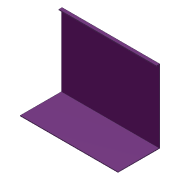
# Autodesk Inventor part: BatteryMount
Saved by Autodesk Inventor 2012 (Build 160160000, 160)
## iProperties
Created: 2013-02-01
Part Number: BatteryMount
Material: Aluminum-6061
Document SubType Name: Modeling
Designer: JesseK
Density: 2.71 g/cm^3
Mass: 290.438 g
Surface Area: 1372.17 cm^2
Volume: 107.173 cm^3
Author: JesseK
Autodesk Inventor part; units mm, degrees
ref_plane "YZ Plane" through (0, 0, 0) normal (1, 0, 0) x (0, 1, 0)
ref_plane "XZ Plane" through (0, 0, 0) normal (0, 1, 0) x (-1, 0, 0)
ref_plane "XY Plane" through (0, 0, 0) normal (0, 0, 1) x (1, 0, 0)
sketch "Sketch1" plane through (0, 0, 0) normal (1, 0, 0) x (0, 1, 0)
  line L0 (1.5875, 103.1875) -> (1.5875, 1.5875)
  line L1 (1.5875, 1.5875) -> (179.3875, 1.5875)
  line L2 (179.3875, 1.5875) -> (179.3875, 7.9375)
  line L3 (179.3875, 7.9375) -> (180.975, 7.9375)
  line L4 (180.975, 7.9375) -> (180.975, 0)
  line L5 (180.975, 0) -> (0, 0)
  line L6 (0, 0) -> (0, 103.1875)
  line L7 (0, 103.1875) -> (1.5875, 103.1875)
  dimension "d0" = 1.5875
  dimension "d1" = 1.5875
  dimension "d2" = 180.975
  dimension "d3" = 101.6
  dimension "d4" = 6.35
  constraints: 16 end point, 4 horizontal, 4 vertical, 1 parallel
  measures "d0" distance between parallel lines of L5 L1
  measures "d1" distance of L2.end L3.end
  measures "d2" distance of L4.end L5.end
  measures "d3" distance of L0.start L0.end
  measures "d4" distance of L1.end L2.end
extrude "Extrusion1" add sketch "Sketch1" along normal blind 241.3
sketch "Sketch2" plane through (0, 0, 0) normal (0, 0, -1) x (-1, 0, 0)
  line L0 (-241.3, 180.975) -> (-241.3, 0) projected
  line L1 (0, 0) -> (-241.3, 0) projected
  line L2 (0, 0) -> (0, 180.975) projected
  line L3 (-241.3, 127) -> (-215.9, 127)
  line L4 (-215.9, 127) -> (-215.9, 76.2)
  line L5 (-215.9, 76.2) -> (-241.3, 76.2)
  line L6 (-241.3, 76.2) -> (-241.3, 127)
  line L7 (0, 127) -> (-25.4, 127)
  line L8 (-25.4, 127) -> (-25.4, 76.2)
  line L9 (-25.4, 76.2) -> (0, 76.2)
  line L10 (0, 76.2) -> (0, 127)
  dimension "d7" = 25.4
  dimension "d8" = 50.8
  dimension "d9" = 76.2
  constraints: 16 end point, 4 parallel, 2 equal length, 2 horizontal, 2 perpendicular, 2 point on line, 1 collinear
  measures "d7" distance of L4.end L5.end
  measures "d8" distance of L3.end L4.end
  measures "d9" distance between parallel lines of L1 L5
extrude "Extrusion2" cut sketch "Sketch2" against normal up to next
sketch "Sketch3" plane through (0, 1.5875, 1.5875) normal (0, 0, 1) x (1, 0, 0)
  line L0 (0, 125.4125) -> (25.4, 125.4125) projected
  line L1 (241.3, 74.6125) -> (215.9, 74.6125) projected
  line L2 (215.9, 125.4125) -> (214.3125, 125.4125)
  line L3 (214.3125, 125.4125) -> (214.3125, 74.6125)
  line L4 (214.3125, 74.6125) -> (215.9, 74.6125)
  line L5 (215.9, 74.6125) -> (215.9, 125.4125)
  line L6 (25.4, 74.6125) -> (26.9875, 74.6125)
  line L7 (26.9875, 74.6125) -> (26.9875, 125.4125)
  line L8 (26.9875, 125.4125) -> (25.4, 125.4125)
  line L9 (25.4, 125.4125) -> (25.4, 74.6125)
  point P0 (0, -1.5875)
  dimension "d12" = 1.5875
  constraints: 16 end point, 4 parallel, 3 collinear, 2 horizontal, 2 perpendicular
  measures "d12" distance of L3.end L4.end
extrude "Extrusion3" add sketch "Sketch3" along normal blind 25.4
sketch "Sketch4" plane through (0, 179.3875, 1.5875) normal (0, 0, 1) x (1, 0, 0)
  line L0 (0, 0) -> (0, -52.3875) projected
  line L1 (241.3, -177.8) -> (241.3, -103.1875) projected
  circle A0 centre (228.6, -23.8125) radius 3.1877
  circle A1 centre (228.6, -125.4125) radius 3.1877
  circle A2 centre (12.7, -23.8125) radius 3.1877
  circle A3 centre (12.7, -125.4125) radius 3.1877
  line L2 (12.7, -23.8125) -> (228.6, -23.8125) construction
  line L3 (228.6, -23.8125) -> (228.6, -125.4125) construction
  line L4 (228.6, -125.4125) -> (12.7, -125.4125) construction
  line L5 (12.7, -125.4125) -> (12.7, -23.8125) construction
  line L6 (0, -179.3875) -> (241.3, -179.3875) construction
  line L7 (0, 1.5875) -> (241.3, 1.5875) construction
  dimension "d15" = 6.3754
  dimension "d16" = 12.7
  dimension "d18" = 25.4
  dimension "d19" = 101.6
  dimension "d20" = 12.7
  constraints: 8 end point, 4 centre point, 3 equal radius, 2 coincident, 2 parallel, 1 horizontal, 1 perpendicular
  measures "d15" diameter of A1
  measures "d16" distance between parallel lines of L0 L5
  measures "d18" distance between parallel lines of L7 L2
  measures "d19" distance of L4.end L2.start
  measures "d20" distance between parallel lines of L1 L3
extrude "Extrusion4" cut sketch "Sketch4" against normal through all
sketch "Sketch5" plane through (0, 0, 0) normal (0, -1, 0) x (1, 0, 0)
  line L0 (0, 103.1875) -> (31.75, 103.1875)
  line L1 (31.75, 103.1875) -> (31.75, 71.4375)
  line L2 (31.75, 71.4375) -> (0, 71.4375)
  line L3 (0, 71.4375) -> (0, 103.1875)
  line L4 (241.3, 103.1875) -> (209.55, 103.1875)
  line L5 (209.55, 103.1875) -> (209.55, 71.4375)
  line L6 (209.55, 71.4375) -> (241.3, 71.4375)
  line L7 (241.3, 71.4375) -> (241.3, 103.1875)
  dimension "d23" = 31.75
  constraints: 16 end point, 4 parallel, 3 equal length, 2 horizontal, 2 perpendicular
  measures "d23" distance between parallel lines of L3 L1
extrude "Extrusion5" cut sketch "Sketch5" against normal up to next
sketch "Sketch6" plane through (0, 1.5875, 1.5875) normal (0, 1, 0) x (1, 0, 0)
  line L0 (209.55, -101.6) -> (209.55, -69.85) projected
  line L1 (31.75, -69.85) -> (31.75, -101.6) projected
  line L2 (31.75, -101.6) -> (209.55, -101.6) projected
  circle A0 centre (76.2, -88.9) radius 3.175
  circle A1 centre (165.1, -88.9) radius 3.175
  line L3 (165.1, -88.9) -> (209.55, -88.9) construction
  line L4 (76.2, -88.9) -> (31.75, -88.9) construction
  point P0 (0, 1.5875)
  dimension "d26" = 12.7
  dimension "d27" = 12.7
  dimension "d28" = 88.9
  dimension "d29" = 6.35
  constraints: 4 end point, 2 centre point, 2 horizontal, 2 point on line, 1 collinear, 1 equal radius
  measures "d26" distance from line of L2 L4.start
  measures "d27" distance from line of L2 L3.start
  measures "d28" distance of L3.start L4.start
  measures "d29" diameter of A1
extrude "Extrusion6" cut sketch "Sketch6" against normal up to next
body "Solid1"
